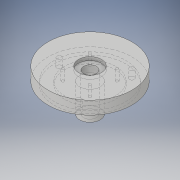
# Autodesk Inventor part: Grabber Base
Saved by Autodesk Inventor 2019.4 (Build 234330000, 330)
## iProperties
Created: 2020-12-03
Part Number: Grabber Base
Material: Generic
Document SubType Name: Modeling
Designer: caleb
Density: 1 g/cm^3
Appearance: Default
Author: caleb
Autodesk Inventor part; units mm, degrees
ref_plane "YZ Plane" through (0, 0, 0) normal (1, 0, 0) x (0, 1, 0)
ref_plane "XZ Plane" through (0, 0, 0) normal (0, 1, 0) x (-1, 0, 0)
ref_plane "XY Plane" through (0, 0, 0) normal (0, 0, 1) x (1, 0, 0)
sketch "Sketch1" plane through (0, 0, 0) normal (0, 1, 0) x (-1, 0, 0)
  circle A0 centre (0, 0) radius 25.98
  dimension "d0" = 51.96
  constraints: 1 centre point, 1 coincident
  measures "d0" diameter of A0
extrude "Extrusion1" add sketch "Sketch1" along normal blind 9.97
sketch "Sketch4" plane through (0, 0, 0) normal (0, -1, 0) x (1, 0, 0)
  circle A0 centre (0, 0) radius 22.21
  circle A1 centre (0, 0) radius 25.98 projected
  dimension "d18" = 44.42
  constraints: 1 centre point, 1 coincident
  measures "d18" diameter of A0
extrude "Extrusion3" cut sketch "Sketch4" against normal blind 1.91
sketch "Sketch6" plane through (0, 0, 0) normal (0, -1, 0) x (1, 0, 0)
  circle A0 centre (0, 0) radius 19
  circle A1 centre (-19, 0) radius 1.525
  circle A2 centre (9.5, -16.4545) radius 1.525
  circle A3 centre (9.5, 16.4545) radius 1.525
  dimension "d21" = 38
  dimension "d22" = 3.05
  dimension "d24" = 19
  dimension "d27" = 360
  constraints: 3 centre point, 1 coincident, 1 horizontal alignment, 9 other
  measures "d22" diameter of A1
  measures "d24" distance of point (0, 0) A1.centre
hole "Hole2" at (-19, 0, 0) at (9.5, 0, 16.4545) at (9.5, 0, -16.4545) direction (0, 1, 0) diameter 3.05 depth 5 tip angle 118
sketch "Sketch9" plane through (0, 0, 0) normal (0, -1, 0) x (1, 0, 0)
  circle A0 centre (0, 0) radius 15.8623
  dimension "d53" = 31.7246
  constraints: 1 centre point, 1 coincident
  measures "d53" diameter of A0
extrude "Extrusion5" cut sketch "Sketch9" against normal blind 1.91
sketch "Sketch10" plane through (0, 1.91, 0) normal (0, -1, 0) x (1, 0, 0)
  circle A0 centre (0, 0) radius 6.3373
  dimension "d56" = 12.6746
  constraints: 1 centre point, 1 coincident
  measures "d56" diameter of A0
extrude "Extrusion6" add sketch "Sketch10" along normal blind 17.7292
sketch "Sketch11" plane through (0, -15.8192, 0) normal (0, -1, 0) x (1, 0, 0)
  circle A0 centre (0, 0) radius 3.9751
  dimension "d59" = 7.9502
  constraints: 1 centre point, 1 coincident
  measures "d59" diameter of A0
extrude "Extrusion7" cut sketch "Sketch11" against normal through all
sketch "Sketch12" plane through (0, 9.97, 0) normal (0, 1, 0) x (1, 0, 0)
  circle A0 centre (0, 0) radius 7.1374
  dimension "d62" = 14.2748
  constraints: 1 centre point, 1 coincident
  measures "d62" diameter of A0
extrude "Extrusion8" cut sketch "Sketch12" against normal blind 2.1336
sketch "Sketch13" plane through (0, 1.91, 0) normal (0, -1, 0) x (1, 0, 0)
  circle A0 centre (0, 0) radius 11.8999
  circle A1 centre (-8.4144, -8.4146) radius 0.889
  circle A2 centre (8.4146, -8.4144) radius 0.889
  circle A3 centre (8.4144, 8.4146) radius 0.889
  circle A4 centre (-8.4146, 8.4144) radius 0.889
  dimension "d65" = 23.7998
  dimension "d66" = 1.778
  dimension "d67" = 8.4146
  dimension "d70" = 360
  constraints: 4 centre point, 1 coincident, 12 other
  measures "d66" diameter of A1
  measures "d67" vertical distance of point (0, 0) A1.centre
hole "Hole4" at (8.4144, 1.91, 8.4146) at (8.4146, 1.91, -8.4144) at (-8.4146, 1.91, 8.4144) at (-8.4144, 1.91, -8.4146) direction (0, 1, 0) diameter 1.694 depth 6.637 tip angle 118 thread size "2-56 UNC" class "2B" standard "ANSI Unified Screw Threads"
body "Solid1"
